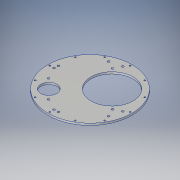
# Autodesk Inventor part: mini 55K stage
Saved by Autodesk Inventor 2018 (Build 220112000, 112)
## iProperties
Created: 2018-10-16
Part Number: mini 55K stage
Material: Aluminum 6061
Document SubType Name: Modeling
Designer: freyja
Density: 2.7 g/cm^3
Appearance: Aluminum - Flat
Mass: 738.698 g
Surface Area: 984.046 cm^2
Volume: 273.592 cm^3
Author: freyja
Autodesk Inventor part; units mm, degrees
ref_plane "YZ Plane" through (0, 0, 0) normal (1, 0, 0) x (0, 1, 0)
ref_plane "XZ Plane" through (0, 0, 0) normal (0, 1, 0) x (-1, 0, 0)
ref_plane "XY Plane" through (0, 0, 0) normal (0, 0, 1) x (1, 0, 0)
sketch "Sketch2" plane through (0, 0, 0) normal (0, 1, 0) x (-1, 0, 0)
  line L0 (0, 0) -> (-28.0184, -28.0184) construction
  line L1 (0, 0) -> (-39.624, 0) construction
  circle A0 centre (-28.0184, -28.0184) radius 139.7
  dimension "d6" = 39.624
  dimension "d7" = 315
  dimension "d8" = 279.4
  constraints: 4 end point, 1 centre point, 1 coincident, 1 equal length, 1 horizontal
  measures "d6" distance of L0.start L0.end
  measures "d8" diameter of A0
extrude "Extrusion1" add sketch "Sketch2" against normal blind 6.35
sketch "Sketch1" plane through (0, 0, 0) normal (0, 1, 0) x (-1, 0, 0)
  line L0 (0, 0) -> (-64.6578, -64.6578) construction
  line L1 (0, 0) -> (91.44, 0) construction
  circle A0 centre (-64.6578, -64.6578) radius 69.85
  line L2 (0, 0) -> (40.4112, 40.4112) construction
  line L3 (0, 0) -> (57.15, 0) construction
  circle A1 centre (40.4112, 40.4112) radius 26.67
  dimension "d0" = 91.44
  dimension "d1" = 135
  dimension "d2" = 139.7
  dimension "d3" = 57.15
  dimension "d4" = 45
  dimension "d5" = 53.34
  constraints: 8 end point, 2 centre point, 2 coincident, 2 equal length, 2 horizontal
  measures "d0" distance of L0.start L0.end
  measures "d1" angle of L0 L1
  measures "d2" diameter of A0
  measures "d3" distance of L0.start L2.end
  measures "d4" angle of L3 L2
  measures "d5" diameter of A1
extrude "Extrusion2" cut sketch "Sketch1" against normal up to surface (6.35 mm away)
sketch "Sketch5" plane through (0, 0, 0) normal (0, 1, 0) x (-1, 0, 0)
  line L0 (0, 0) -> (0, -165.1) construction
  line L1 (0, 0) -> (165.1, 0) construction
  line L2 (0, -165.1) -> (-17.9605, -147.1395)
  line L3 (0, 0) -> (-165.1, 0) construction
  line L4 (0, 0) -> (165.1, 0) construction
  line L5 (-165.1, 0) -> (-147.1395, -17.9605)
  line L6 (0, 0) -> (-28.0184, -28.0184) construction
  line L7 (0, 0) -> (39.624, 0) construction
  line L8 (-28.0184, -28.0184) -> (91.514, -28.0184)
  line L9 (-28.0184, -28.0184) -> (91.514, -28.0184) construction
  line L10 (-28.0184, -28.0184) -> (-28.0184, 91.514)
  line L11 (-28.0184, -28.0184) -> (91.514, -28.0184) construction
  dimension "d44" = 165.1
  dimension "d45" = 90
  dimension "d46" = 25.4
  dimension "d47" = 45
  dimension "d48" = 165.1
  dimension "d49" = 180
  dimension "d50" = 25.4
  dimension "d51" = 45
  dimension "d52" = 39.624
  dimension "d53" = 135
  dimension "d54" = 119.5324
  dimension "d55" = 0
  dimension "d56" = 119.5324
  dimension "d57" = 90
  constraints: 24 end point, 6 horizontal, 5 equal length, 2 vertical, 1 perpendicular
  measures "d44" distance of L0.start L0.end
  measures "d45" angle of L0 L1
  measures "d46" distance of L0.end L2.end
  measures "d47" angle of L0 L2
  measures "d48" distance of L0.start L3.end
  measures "d49" angle of L3 L4
  measures "d50" distance of L3.end L5.end
  measures "d51" angle of L5 L3
  measures "d52" distance of L0.start L6.end
  measures "d53" angle of L6 L7
  measures "d54" distance of L6.end L8.end
  measures "d55" distance between parallel lines of L8 L9
  measures "d56" distance of L6.end L10.end
  measures "d57" angle of L11 L10
hole "Hole2" at (28.0184, 0, 91.514) at (-91.514, 0, -28.0184) at (17.9605, 0, -147.1395) at (147.1395, 0, -17.9605) direction (0, -1, 0) diameter 4.9784 end through all thread size "1/4-20 UNC" class "2B" standard "ANSI Unified Screw Threads"
sketch "Sketch6" plane through (28.0184, 0, -28.0184) normal (0, 1, 0) x (1, 0, 0)
  circle A0 centre (0, 0) radius 139.7 projected
  line L0 (0, 0) -> (115.4845, 66.675)
  line L1 (0, 0) -> (133.35, 0) construction
  point P0 (-28.0184, -28.0184)
  dimension "d65" = 133.35
  dimension "d66" = 30
  constraints: 4 end point, 1 equal length, 1 horizontal
  measures "d65" distance of L0.start L0.end
  measures "d66" angle of L1 L0
hole "Hole3" at (143.5029, 0, -94.6934) direction (0, -1, 0) diameter 4.9784 end through all thread size "1/4-20 UNC" class "2B" standard "ANSI Unified Screw Threads"
pattern_circular "Circular Pattern1" count 12 over 360 about axis through (28.0184, 0, -28.0184) along (0, -1, 0) of "Hole3"
sketch "Sketch11" plane through (28.0184, 0, -28.0184) normal (0, 1, 0) x (1, 0, 0)
  line L0 (-28.0184, -28.0184) -> (137.3706, 110.7594) construction
  line L1 (-28.0184, -28.0184) -> (187.8816, -28.0184) construction
  line L2 (-28.0184, -28.0184) -> (110.7594, 137.3706) construction
  line L3 (-28.0184, -28.0184) -> (187.8816, -28.0184) construction
  circle A0 centre (137.3706, 110.7594) radius 122.1994
  circle A1 centre (110.7594, 137.3706) radius 122.1994
  circle A2 centre (-166.7962, 137.3706) radius 122.1994
  circle A3 centre (-193.4074, 110.7594) radius 122.1994
  circle A4 centre (-193.4074, -166.7962) radius 122.1994
  circle A5 centre (-166.7962, -193.4074) radius 122.1994
  circle A6 centre (110.7594, -193.4074) radius 122.1994
  circle A7 centre (137.3706, -166.7962) radius 122.1994
  line L4 (0, 0) -> (196.85, 0) construction
  circle A8 centre (0, 0) radius 139.7 projected
  line L5 (0, 0) -> (-150.7958, -126.5327)
  line L6 (0, 0) -> (196.85, 0) construction
  line L7 (0, 0) -> (-126.5327, -150.7958)
  line L8 (0, 0) -> (196.85, 0) construction
  circle A9 centre (-150.7958, -126.5327) radius 130.3378
  circle A10 centre (-126.5327, -150.7958) radius 130.3378
  circle A11 centre (0, 0) radius 119.5449
  circle A12 centre (119.1211, -10.0579) radius 2.4892 projected
  circle A13 centre (-119.5324, 0) radius 2.4892 projected
  circle A14 centre (0, -119.5324) radius 2.4892 projected
  point P0 (118.5463, 15.4195)
  point P1 (109.5723, -47.8007)
  point P2 (14.043, -118.7173)
  point P3 (0.0031, -119.5449)
  point P4 (-119.5449, 0.0031)
  point P5 (-118.7173, 14.043)
  point P6 (-47.8007, 109.5723)
  point P7 (-10.0694, 119.1201)
  point P8 (119.1201, -10.0694)
  dimension "d101" = 244.3988
  dimension "d123" = 239.0899
  dimension "d97" = 215.9
  dimension "d98" = 40
  dimension "d99" = 215.9
  dimension "d100" = 50
  dimension "d102" = 244.3988
  dimension "d105" = 360
  dimension "d109" = 196.85
  dimension "d110" = 140
  dimension "d111" = 196.85
  dimension "d112" = 130
  dimension "d124" = 260.6756
  constraints: 18 end point, 8 coincident, 6 point on circle, 5 centre point, 5 horizontal, 4 equal length, 44 other
  measures "d97" distance of L0.start L0.end
  measures "d98" angle of L1 L0
  measures "d99" distance of L0.start L2.end
  measures "d100" angle of L3 L2
  measures "d102" diameter of A1
  measures "d109" distance of L5.start L5.end
  measures "d110" angle of L5 L6
  measures "d111" distance of L5.start L7.end
  measures "d112" angle of L7 L8
  measures "d124" diameter of A9
hole "Hole5" at (-90.6989, 0, -42.0614) at (137.5907, 0, 19.7823) at (-19.7823, 0, -137.5907) at (17.949, 0, -147.1385) at (147.1385, 0, -17.949) at (42.0614, 0, 90.6989) at (-91.5265, 0, -28.0215) at (28.0215, 0, 91.5265) direction (0, -1, 0) diameter 6.7564 end through all clearance for "Flat Head Machine Screw (82)" size "1/4" standard "Ansi Unified Screw Threads"
sketch "Sketch12" plane through (28.0184, 0, -28.0184) normal (0, 1, 0) x (1, 0, 0)
  circle A0 centre (0, 0) radius 139.7 projected
  line L0 (-28.0184, -28.0184) -> (-3.7717, -3.7717)
  line L1 (-28.0184, -28.0184) -> (6.2716, -28.0184) construction
  line L2 (-3.7717, -3.7717) -> (-21.4144, 96.2848)
  line L3 (-3.7717, -3.7717) -> (97.8283, -3.7717) construction
  line L4 (-3.7717, -3.7717) -> (-99.2445, -38.521)
  line L5 (-3.7717, -3.7717) -> (97.8283, -3.7717) construction
  line L6 (-3.7717, -3.7717) -> (14.1888, 14.1888)
  line L7 (-3.7717, -3.7717) -> (21.6283, -3.7717) construction
  line L8 (-3.7717, -3.7717) -> (96.2848, -21.4144)
  line L9 (-3.7717, -3.7717) -> (-38.521, -99.2445)
  point P0 (96.2848, -21.4144)
  point P1 (-38.521, -99.2445)
  dimension "d139" = 34.29
  dimension "d140" = 45
  dimension "d141" = 101.6
  dimension "d142" = 100
  dimension "d143" = 101.6
  dimension "d144" = 160
  dimension "d145" = 25.4
  dimension "d146" = 45
  constraints: 20 end point, 4 coincident, 4 equal length, 4 horizontal, 2 symmetric about line
  measures "d139" distance of L0.start L0.end
  measures "d140" angle of L1 L0
  measures "d141" distance of L0.end L2.end
  measures "d142" angle of L3 L2
  measures "d143" distance of L0.end L4.end
  measures "d144" angle of L4 L5
  measures "d145" distance of L0.end L6.end
  measures "d146" angle of L7 L6
hole "Hole6" at (6.604, 0, -124.3032) at (-71.2261, 0, 10.5026) at (-10.5026, 0, 71.2261) at (124.3032, 0, -6.604) direction (0, -1, 0) diameter 6.7564 end through all clearance for "Flat Head Machine Screw (82)" size "1/4" standard "Ansi Unified Screw Threads"
body "Solid1"
